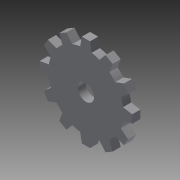
# Autodesk Inventor part: Sun
Saved by Autodesk Inventor 2013 (Build 170138000, 138)
## iProperties
Created: 2014-02-12
Part Number: Sun
Material: Generic
Document SubType Name: Modeling
Designer: robotics
Density: 1 g/cm^3
Author: robotics
Autodesk Inventor part; units mm, degrees
ref_plane "YZ Plane" through (0, 0, 0) normal (1, 0, 0) x (0, 1, 0)
ref_plane "XZ Plane" through (0, 0, 0) normal (0, 1, 0) x (-1, 0, 0)
ref_plane "XY Plane" through (0, 0, 0) normal (0, 0, 1) x (1, 0, 0)
sketch "Sketch2" plane through (0, 0, 0) normal (0, 0, 1) x (1, 0, 0)
  line L0 (0, 15.4964) -> (0, 0) construction
  line L1 (1.1069, 7.1978) -> (0.7937, 8.9739)
  line L2 (0.7937, 8.9739) -> (0, 8.9739)
  line L3 (-1.1069, 7.1978) -> (-0.7937, 8.9739)
  line L4 (-0.7937, 8.9739) -> (0, 8.9739)
  line L5 (-2.6403, 6.787) -> (-3.7995, 8.1685)
  line L6 (-3.7995, 8.1685) -> (-4.4869, 7.7716)
  line L7 (-4.5575, 5.6801) -> (-5.1743, 7.3747)
  line L8 (-5.1743, 7.3747) -> (-4.4869, 7.7716)
  line L9 (-5.6801, 4.5575) -> (-7.3747, 5.1743)
  line L10 (-7.3747, 5.1743) -> (-7.7716, 4.4869)
  line L11 (-6.787, 2.6403) -> (-8.1685, 3.7995)
  line L12 (-8.1685, 3.7995) -> (-7.7716, 4.4869)
  line L13 (-7.1978, 1.1069) -> (-8.9739, 0.7938)
  line L14 (-8.9739, 0.7938) -> (-8.9739, 0)
  line L15 (-7.1978, -1.1069) -> (-8.9739, -0.7937)
  line L16 (-8.9739, -0.7937) -> (-8.9739, 0)
  line L17 (-6.787, -2.6403) -> (-8.1685, -3.7995)
  line L18 (-8.1685, -3.7995) -> (-7.7716, -4.4869)
  line L19 (-5.6801, -4.5575) -> (-7.3747, -5.1743)
  line L20 (-7.3747, -5.1743) -> (-7.7716, -4.4869)
  line L21 (-4.5575, -5.6801) -> (-5.1743, -7.3747)
  line L22 (-5.1743, -7.3747) -> (-4.4869, -7.7716)
  line L23 (-2.6403, -6.787) -> (-3.7995, -8.1685)
  line L24 (-3.7995, -8.1685) -> (-4.4869, -7.7716)
  line L25 (-1.1069, -7.1978) -> (-0.7938, -8.9739)
  line L26 (-0.7938, -8.9739) -> (0, -8.9739)
  line L27 (1.1069, -7.1978) -> (0.7937, -8.9739)
  line L28 (0.7937, -8.9739) -> (0, -8.9739)
  line L29 (2.6403, -6.787) -> (3.7995, -8.1685)
  line L30 (3.7995, -8.1685) -> (4.4869, -7.7716)
  line L31 (4.5575, -5.6801) -> (5.1743, -7.3747)
  line L32 (5.1743, -7.3747) -> (4.4869, -7.7716)
  line L33 (5.6801, -4.5575) -> (7.3747, -5.1743)
  line L34 (7.3747, -5.1743) -> (7.7716, -4.4869)
  line L35 (6.787, -2.6403) -> (8.1685, -3.7995)
  line L36 (8.1685, -3.7995) -> (7.7716, -4.4869)
  line L37 (7.1978, -1.1069) -> (8.9739, -0.7938)
  line L38 (8.9739, -0.7938) -> (8.9739, 0)
  line L39 (7.1978, 1.1069) -> (8.9739, 0.7937)
  line L40 (8.9739, 0.7937) -> (8.9739, 0)
  line L41 (6.787, 2.6403) -> (8.1685, 3.7995)
  line L42 (8.1685, 3.7995) -> (7.7716, 4.4869)
  line L43 (5.6801, 4.5575) -> (7.3747, 5.1743)
  line L44 (7.3747, 5.1743) -> (7.7716, 4.4869)
  line L45 (4.5575, 5.6801) -> (5.1743, 7.3747)
  line L46 (5.1743, 7.3747) -> (4.4869, 7.7716)
  line L47 (2.6403, 6.787) -> (3.7995, 8.1685)
  line L48 (3.7995, 8.1685) -> (4.4869, 7.7716)
  line L49 (-2.6403, 6.787) -> (-1.1069, 7.1978) construction
  line L50 (-0.7937, 8.9739) -> (0.7937, 8.9739) construction
  arc A0 (-1.1069, 7.1978) -> (-2.6403, 6.787) centre (0, 0) ccw
  arc A1 (-4.5575, 5.6801) -> (-5.6801, 4.5575) centre (0, 0) ccw
  arc A2 (-6.787, 2.6403) -> (-7.1978, 1.1069) centre (0, 0) ccw
  arc A3 (-7.1978, -1.1069) -> (-6.787, -2.6403) centre (0, 0) ccw
  arc A4 (-5.6801, -4.5575) -> (-4.5575, -5.6801) centre (0, 0) ccw
  arc A5 (-2.6403, -6.787) -> (-1.1069, -7.1978) centre (0, 0) ccw
  arc A6 (1.1069, -7.1978) -> (2.6403, -6.787) centre (0, 0) ccw
  arc A7 (4.5575, -5.6801) -> (5.6801, -4.5575) centre (0, 0) ccw
  arc A8 (6.787, -2.6403) -> (7.1978, -1.1069) centre (0, 0) ccw
  arc A9 (7.1978, 1.1069) -> (6.787, 2.6403) centre (0, 0) ccw
  arc A10 (5.6801, 4.5575) -> (4.5575, 5.6801) centre (0, 0) ccw
  arc A11 (2.6403, 6.787) -> (1.1069, 7.1978) centre (0, 0) ccw
  line L51 (0, 0) -> (3.0862, 0) construction
  dimension "d5" = 1.5875
  dimension "d13" = 1.8034
  dimension "d14" = 100
  constraints: 104 end point, 24 point on circle, 12 centre point, 2 symmetric about line, 1 coincident, 1 collinear, 1 equal length, 1 parallel, 1 perpendicular, 1 point on line, 1 vertical, 109 other
  measures "d5" distance of L3.end L1.end
  measures "d13" distance of L1.start L1.end
  measures "d14" angle of L51 L1
extrude "Extrusion1" add sketch "Sketch2" along normal blind 1.5875
sketch "Sketch3" plane through (0, 0, 1.5875) normal (0, 0, 1) x (1, 0, 0)
  arc A0 (2.6403, 6.787) -> (1.1069, 7.1978) centre (0, 0) ccw projected
  circle A1 centre (0, 0) radius 1.5875
  dimension "d10" = 3.175
  constraints: 1 centre point, 1 coincident
  measures "d10" diameter of A1
extrude "Extrusion2" cut sketch "Sketch3" against normal up to next
body "Solid1"
